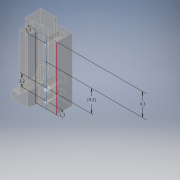
# Autodesk Inventor part: Top
Saved by Autodesk Inventor 2020 (Build 240168000, 168)
## iProperties
Created: 2019-02-07
Part Number: Top
Material: 유리
Document SubType Name: Modeling
Designer: Jeong Ji Hoon
Density: 2.18 g/cm^3
Appearance: 연회색 반사
Author: Jeong Ji Hoon
## iProperties of the stored document _3D 인쇄.ipt
Created: 2019-11-29
Part Number: _3D 인쇄
Material: 일반
Document SubType Name: Modeling
Designer: Knowblesse
Density: 1 g/cm^3
Appearance: 기본값
Author: Knowblesse
Autodesk Inventor part; units mm, degrees
ref_plane "YZ Plane" through (0, 0, 0) normal (1, 0, 0) x (0, 1, 0)
ref_plane "XZ Plane" through (0, 0, 0) normal (0, 1, 0) x (-1, 0, 0)
ref_plane "XY Plane" through (0, 0, 0) normal (0, 0, 1) x (1, 0, 0)
sketch "스케치1" plane through (0, 0, 0) normal (0, 0, 1) x (1, 0, 0)
  line L0 (0, 0) -> (4, 0)
  line L1 (4, 0) -> (4, 12)
  line L2 (4, 12) -> (0, 12)
  line L3 (0, 12) -> (0, 0)
  dimension "d0" = 4
  dimension "d1" = 12
  constraints: 8 end point, 2 parallel, 1 horizontal, 1 perpendicular
  measures "d0" distance of L2.end L1.end
  measures "d1" distance of L1.end L0.end
extrude "돌출1" add sketch "스케치1" along normal blind 3
sketch "스케치2" plane through (0, 0, 3) normal (0, 0, 1) x (1, 0, 0)
  line L0 (4, 12) -> (0, 12) construction
  line L1 (2, 12) -> (2, 0) construction
  line L2 (0, 0) -> (4, 0) construction
  line L3 (4, 0) -> (4, 12) projected
  line L4 (0, 12) -> (0, 0) projected
  point P0 (2, 7.7)
  point P1 (2, 3.5)
  point P2 (2, 1.3)
  point P3 (2, 10.7)
  dimension "d9" = 4.3
  dimension "d45" = 1.3
  dimension "d51" = 4.2
  dimension "d52" = 2.2
  dimension "d55" = 1.3
  constraints: 4 point on line, 2 end point, 2 midpoint
  measures "d9" distance from line of L0 point (2, 7.7)
  measures "d45" distance from line of point (2, 1.3) L2
  measures "d51" distance of point (2, 3.5) point (2, 7.7)
  measures "d52" distance of point (2, 1.3) point (2, 3.5)
  measures "d55" distance from line of point (2, 10.7) L0
hole "구멍2" at (2, 3.5, 3) direction (0, 0, -1) diameter 1.6 end through all
hole "구멍3" at (2, 1.3, 3) at (2, 10.7, 3) direction (0, 0, -1) diameter 1 end through all
sketch "스케치5" plane through (0, 0, 0) normal (-1, 0, 0) x (0, 0, 1)
  line L0 (0, 12) -> (0, 0) projected
  line L1 (0, 0) -> (3, 0) projected
  line L2 (3, 12) -> (3, 0) projected
  line L3 (0, 12) -> (3, 12) projected
  line L4 (-1, 12) -> (4.5, 12)
  line L5 (4.5, 12) -> (4.5, 0)
  line L6 (4.5, 0) -> (-1, 0)
  line L7 (-1, 0) -> (-1, 12)
  line L8 (0, 0) -> (3, 0) projected
  dimension "d62" = 4.5
  dimension "d71" = 1
  constraints: 8 end point, 2 collinear, 2 parallel, 1 horizontal
  measures "d62" distance between parallel lines of L5 L0
  measures "d71" distance between parallel lines of L0 L7
extrude "돌출5" add sketch "스케치5" along normal blind 2
sketch "스케치6" plane through (-2, 0, 0) normal (-1, 0, 0) x (0, 0, 1)
  line L0 (4.5, 0) -> (4.5, 12) projected
  line L1 (4.5, 12) -> (-1, 12) projected
  line L2 (-1, 12) -> (-1, 0) projected
  line L3 (-1, 0) -> (4.5, 0) projected
  line L4 (4.5, 0) -> (4.5, 12) projected
  line L5 (4.5, 12) -> (-1, 12)
  line L6 (-1, 12) -> (-1, 10.7)
  line L7 (-1, 10.7) -> (4.5, 10.7)
  line L8 (4.5, 10.7) -> (4.5, 12)
  line L9 (-1, 12) -> (-1, 0) projected
  line L10 (-1, 0) -> (4.5, 0)
  line L11 (4.5, 0) -> (4.5, 1.3)
  line L12 (4.5, 1.3) -> (-1, 1.3)
  line L13 (-1, 1.3) -> (-1, 0)
  line L14 (-1, 12) -> (-1, 0) projected
  line L15 (-1, 9.2) -> (0.5, 10.7)
  line L16 (-1, 2.8) -> (0.5, 1.3)
  point P0 (-1, 1.3)
  point P1 (4.5, 10.7)
  dimension "d72" = 9.4
  dimension "d73" = 1.3
  dimension "d74" = 1.3
  dimension "d78" = 1.5
  dimension "d79" = 45
  dimension "d80" = 45
  constraints: 20 end point, 6 point on line, 4 parallel, 2 horizontal, 2 perpendicular, 1 vertical alignment
  measures "d72" distance between parallel lines of L12 L7
  measures "d73" distance between parallel lines of L1 L7
  measures "d74" distance between parallel lines of L3 L12
  measures "d78" distance of L15.end L6.end
  measures "d79" angle of L2 L15
  measures "d80" angle of L2 L16
extrude "돌출6" add sketch "스케치6" along normal blind 1 contours L3 L2 L12 L0 | L7 L2 L1 L0 | L12 L2 L16 | L15 L2 L7
chamfer "모따기2" distance 0.5 angle 45 1 edges at (0, 6, 0)
sketch "스케치7" plane through (-2, 0, 0) normal (-1, 0, 0) x (0, 0, 1)
  line L0 (-1, 2.8) -> (0.5, 1.3) projected
  line L1 (0.5, 1.3) -> (4.5, 1.3) projected
  line L2 (4.5, 1.3) -> (4.5, 10.7) projected
  line L3 (4.5, 10.7) -> (0.5, 10.7) projected
  line L4 (0.5, 10.7) -> (-1, 9.2) projected
  line L5 (-1, 9.2) -> (-1, 2.8) projected
extrude "돌출7" cut sketch "스케치7" against normal blind 0.5
sketch "스케치8" plane through (-3, 1.3, 4.5) normal (0, 1, 0) x (1, 0, 0)
  line L0 (1.5, 4) -> (1.5, 0) projected
  arc A0 (1.5, 1) -> (1.5, 4.5) centre (-4.2391, 2.75) ccw
  line L1 (7, 4.5) -> (3.5, 4.5) projected
  line L2 (3, 5) -> (3.5, 4.5) projected
  line L3 (3, 5) -> (3, 5.5) projected
  line L4 (3, 5.5) -> (0, 5.5) projected
  line L5 (0, 0) -> (0, 5.5) projected
  line L6 (3, 0) -> (0, 0) projected
  line L7 (3, 0) -> (3, 1.5) projected
  line L8 (7, 1.5) -> (3, 1.5) projected
  line L9 (7, 4.5) -> (7, 1.5) projected
  line L10 (1.5, 1) -> (1.5, 4.5)
  line L11 (1.5, 4) -> (1.5, 5.5) projected
  point P0 (3, 4.5)
  point P1 (1.5, 4)
  dimension "d84" = 6
  constraints: 2 end point, 2 point on circle, 2 point on line, 1 centre point, 1 collinear, 1 horizontal alignment
  measures "d84" radius of A0
extrude "돌출8" cut sketch "스케치8" along normal up to surface (9.4 mm away) contours L10 A0 L0
chamfer "모따기3" distance 0.5 distance2 1.5 1 edges at (0, 6, 3) measured on face at (0.5, 6, 3)
sketch "스케치9" plane through (-3, 0, 0) normal (-1, 0, 0) x (0, 0, 1)
  line L0 (-1, 12) -> (-1, 9.2) projected
  line L1 (-1, 9.2) -> (0.5, 10.7) projected
  line L2 (0.5, 10.7) -> (4.5, 10.7) projected
  line L3 (4.5, 10.7) -> (4.5, 12) projected
  line L4 (4.5, 12) -> (-1, 12) projected
  line L5 (2, 12) -> (2, 10.7)
  line L6 (0.5, 10.7) -> (4.5, 10.7) projected
  point P0 (0, 0)
  dimension "d91" = 2.5
  constraints: 2 end point, 2 point on line, 1 perpendicular
  measures "d91" distance between parallel lines of L3 L5
extrude "돌출9" cut sketch "스케치9" against normal up to surface (1.5 mm away) contours L4 L3 L2 L5
equation "\"d73\" = d74"
equation "\"d80\" = d79"
equation "\"G23_M\" = 0.67"
equation "\"G23_F\" = 0.65"
